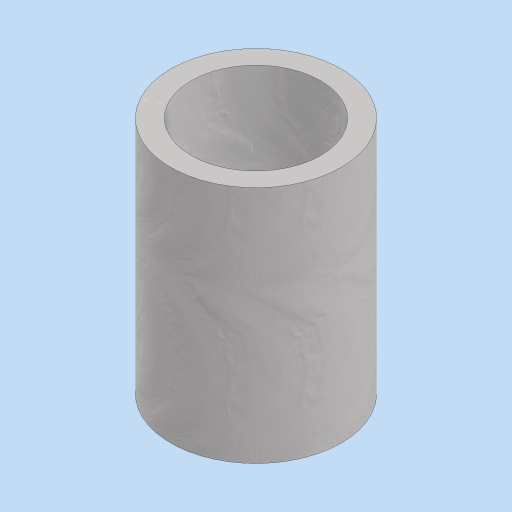
# Autodesk Inventor part: tube
Saved by Autodesk Inventor 2023 (Build 270158000, 158)
## iProperties
Created: 2026-04-08
Part Number: tube
Material: Steel, Mild, Welded
Document SubType Name: Modeling
Designer: Nathann
Density: 7.85 g/cm^3
Appearance: Weld - Steel Mild
Author: Nathann
Autodesk Inventor part; units mm, degrees
ref_plane "YZ Plane" through (0, 0, 0) normal (1, 0, 0) x (0, 1, 0)
ref_plane "XZ Plane" through (0, 0, 0) normal (0, 1, 0) x (-1, 0, 0)
ref_plane "XY Plane" through (0, 0, 0) normal (0, 0, 1) x (1, 0, 0)
sketch "Sketch1" plane through (0, 0, 0) normal (0, 1, 0) x (-1, 0, 0)
  circle A0 centre (0, 0) radius 25
  circle A1 centre (0, 0) radius 19
  dimension "d0" = 50
  dimension "d1" = 38
  constraints: 2 centre point, 2 coincident
  measures "d0" diameter of A0
  measures "d1" diameter of A1
extrude "Extrusion1" add sketch "Sketch1" along normal blind 70
body "Solid1"
